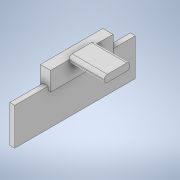
# Autodesk Inventor part: eonPCB
Saved by Autodesk Inventor 2020 (Build 240168000, 168)
## iProperties
Created: 2021-01-18
Part Number: eonPCB
Material: Generic
Document SubType Name: Modeling
Designer: dkiiv
Density: 1 g/cm^3
Appearance: Default
Author: dkiiv
Autodesk Inventor part; units mm, degrees
ref_plane "YZ Plane" through (0, 0, 0) normal (1, 0, 0) x (0, 1, 0)
ref_plane "XZ Plane" through (0, 0, 0) normal (0, 1, 0) x (-1, 0, 0)
ref_plane "XY Plane" through (0, 0, 0) normal (0, 0, 1) x (1, 0, 0)
sketch "Sketch1" plane through (0, 0, 0) normal (0, 1, 0) x (-1, 0, 0)
  line L0 (0, 0) -> (16.8, 0)
  line L1 (16.8, 0) -> (16.8, -39)
  line L2 (16.8, -39) -> (0, -39)
  line L3 (0, -39) -> (0, 0)
  line L4 (16.8, -10.8) -> (10.7, -10.8)
  line L5 (10.7, -10.8) -> (10.7, -31)
  line L6 (10.7, -31) -> (16.8, -31)
  line L7 (16.8, -31) -> (16.8, -10.8)
  line L8 (0, -25.4905) -> (10.7, -25.4905)
  line L9 (10.7, -25.4905) -> (10.7, -14.3627)
  line L10 (10.7, -14.3627) -> (0, -14.3627)
  line L11 (0, -14.3627) -> (0, -25.4905)
  dimension "d0" = 16.8
  dimension "d1" = 39
  dimension "d2" = 6.1
  dimension "d3" = 20.2
  dimension "d4" = 0
  dimension "d5" = 10.7
  dimension "d6" = 8
  constraints: 24 end point, 6 parallel, 3 horizontal, 3 perpendicular, 1 point on line
  measures "d0" distance of L1.end L2.end
  measures "d1" distance of L0.end L1.end
  measures "d2" distance of L6.end L5.end
  measures "d3" distance of L6.end L4.start
  measures "d4" distance between parallel lines of L1 L7
  measures "d5" distance of L10.end L9.end
  measures "d6" distance between parallel lines of L2 L6
extrude "Extrusion1" add sketch "Sketch1" along normal blind 1.6 contours L0 L1 L4 L5 L10 L3 | L10 L5 L8 L3 | L8 L5 L6 L1 L2 L3
extrude "Extrusion2" add sketch "Sketch1" along normal blind 2.4 and the other way blind 0.9 contours L1 L6 L5 L4
sketch "Sketch2" plane through (0, 2.4, 0) normal (0, 1, 0) x (1, 0, 0)
  line L0 (-16.95, 16.75) -> (-16.65, 16.75)
  line L1 (-15.65, 17.75) -> (-15.65, 24.05)
  line L2 (-16.65, 25.05) -> (-16.95, 25.05)
  line L3 (-17.95, 24.05) -> (-17.95, 17.75)
  line L4 (-16.8, 31) -> (-16.8, 10.8) projected
  line L5 (-10.7, 31) -> (-16.8, 31) projected
  line L6 (-16.8, 10.8) -> (-10.7, 10.8) projected
  arc A0 (-16.95, 25.05) -> (-17.95, 24.05) centre (-16.95, 24.05) ccw
  arc A1 (-15.65, 24.05) -> (-16.65, 25.05) centre (-16.65, 24.05) ccw
  arc A2 (-17.95, 17.75) -> (-16.95, 16.75) centre (-16.95, 17.75) ccw
  arc A3 (-16.65, 16.75) -> (-15.65, 17.75) centre (-16.65, 17.75) ccw
  point P0 (0, 0)
  point P1 (-17.95, 16.75)
  point P2 (-15.65, 25.05)
  point P3 (-17.95, 25.05)
  dimension "d13" = 2.3
  dimension "d14" = 8.3
  dimension "d15" = 1.15
  dimension "d16" = 5.95
  dimension "d17" = 5.95
  dimension "d18" = 1
  constraints: 8 end point, 8 point on circle, 8 tangent, 6 point on line, 4 centre point, 3 equal radius, 2 parallel, 1 horizontal, 1 perpendicular
  measures "d13" distance of point (-15.65, 25.05) point (-17.95, 25.05)
  measures "d14" distance of point (-17.95, 25.05) point (-17.95, 16.75)
  measures "d15" distance between parallel lines of L4 L1
  measures "d16" distance between parallel lines of L5 L2
  measures "d17" distance between parallel lines of L6 L0
  measures "d18" radius of A0
extrude "Extrusion3" add sketch "Sketch2" along normal blind 11.4
sketch "Sketch3" plane through (0, 0, 0) normal (0, -1, 0) x (1, 0, 0)
  line L0 (0, 0) -> (0, -39) projected
  line L1 (0, 0) -> (-12, 0)
  line L2 (-12, 0) -> (-12, -10.8)
  line L3 (-12, -10.8) -> (0, -10.8)
  line L4 (0, -10.8) -> (0, 0)
  line L5 (-10.7, -31) -> (-16.8, -31) projected
  line L6 (-12, -31) -> (0, -31)
  line L7 (0, -31) -> (0, -39)
  line L8 (0, -39) -> (-12, -39)
  line L9 (-12, -39) -> (-12, -31)
  line L10 (-16.8, -39) -> (-12, -39)
  line L11 (-12, -39) -> (-12, -31)
  line L12 (-12, -31) -> (-16.8, -31)
  line L13 (-16.8, -31) -> (-16.8, -39)
  line L14 (-16.8, -10.8) -> (-12, -10.8)
  line L15 (-12, -10.8) -> (-12, 0)
  line L16 (-12, 0) -> (-16.8, 0)
  line L17 (-16.8, 0) -> (-16.8, -10.8)
  dimension "d21" = 12
  dimension "d22" = 10.8
  constraints: 32 end point, 8 parallel, 4 horizontal, 4 perpendicular, 1 point on line
  measures "d21" distance of L3.end L2.end
  measures "d22" distance of L1.end L2.end
extrude "Extrusion4" cut sketch "Sketch3" against normal blind 10.1 contours L2 L14 L17 L16 | L10 L13 L5 L9
body "Solid1"
